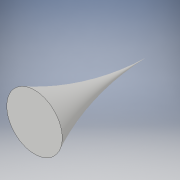
# Autodesk Inventor part: Spike tip
Saved by Autodesk Inventor 2017 (Build 210142000, 142)
## iProperties
Created: 2016-10-16
Part Number: Spike tip
Material: Generic
Document SubType Name: Modeling
Designer: Will
Density: 1 g/cm^3
Appearance: Default
Author: Will
Autodesk Inventor part; units mm, degrees
ref_plane "YZ Plane" through (0, 0, 0) normal (1, 0, 0) x (0, 1, 0)
ref_plane "XZ Plane" through (0, 0, 0) normal (0, 1, 0) x (-1, 0, 0)
ref_plane "XY Plane" through (0, 0, 0) normal (0, 0, 1) x (1, 0, 0)
sketch "Sketch1" plane through (0, 0, 0) normal (0, 1, 0) x (-1, 0, 0)
  line L0 (0, 0) -> (-19.05, 0)
  line L1 (-19.05, 0) -> (-19.05, -76.2)
  arc A0 (0, 0) -> (-19.05, -76.2) centre (159.6547, -80.3949) ccw
  dimension "d0" = 19.05
  dimension "d1" = 76.2
  constraints: 4 end point, 2 point on circle, 1 centre point, 1 horizontal, 1 perpendicular
  measures "d0" distance of L0.start L0.end
  measures "d1" distance of L0.end L1.end
revolve "Revolution1" add sketch "Sketch1" angle 360 about axis through (19.05, 0, 0) along (0, 0, -1)
body "Solid1"
